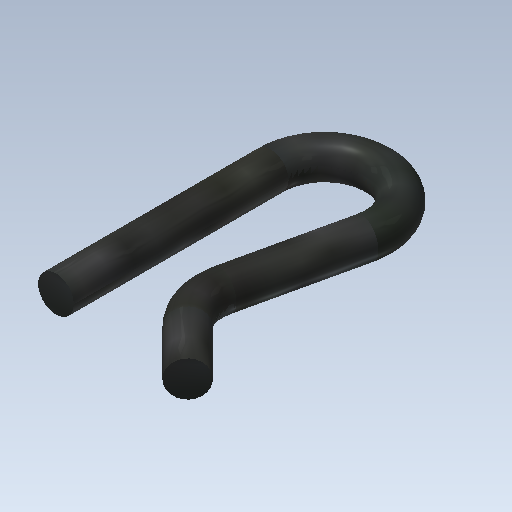
# Autodesk Inventor part: 500-177
Saved by Autodesk Inventor 2020 (Build 240168000, 168)
## iProperties
Created: 2015-04-18
Part Number: 500-177
Material: Steel
Document SubType Name: Modeling
Designer: Station9
Mass: 0.108858 g
Surface Area: 0.5704 cm^2
Volume: 0.0138673 cm^3
Density: 7.85 g/cm^3
Appearance: Plate
Author: Station9
Autodesk Inventor part; units mm, degrees
ref_plane "YZ Plane" through (0, 0, 0) normal (1, 0, 0) x (0, 1, 0)
ref_plane "XZ Plane" through (0, 0, 0) normal (0, 1, 0) x (-1, 0, 0)
ref_plane "XY Plane" through (0, 0, 0) normal (0, 0, 1) x (1, 0, 0)
sketch "Sketch1" plane through (0, 0, 0) normal (0, 1, 0) x (-1, 0, 0)
  line L0 (0, 0) -> (0, -6)
  arc A0 (-1.9758, -5.7812) -> (0, -6) centre (-1, -6) ccw
  line L1 (-1.9758, -5.7812) -> (-1.2485, -2.5376)
  line L2 (-1.7858, -0.6858) -> (-3.0444, 0.5729)
  arc A1 (-1.2485, -2.5376) -> (-1.7858, -0.6858) centre (-3.2, -2.1) ccw
  dimension "d0" = 2
  dimension "d1" = 1
  dimension "d2" = 6
  dimension "d3" = 1.78
  dimension "d4" = 3.9
  dimension "d5" = 2.2
  dimension "d6" = 45
  constraints: 6 end point, 4 point on circle, 4 tangent, 2 centre point, 1 vertical
  measures "d0" radius of A1
  measures "d1" radius of A0
  measures "d2" distance of L0.start L0.end
  measures "d3" distance of L2.start L2.end
  measures "d4" vertical distance of A0.centre A1.centre
  measures "d5" horizontal distance of A0.centre A1.centre
  measures "d6" angle of L0 L2
sketch "Sketch2" plane through (0, 0, 0) normal (0, 0, 1) x (1, 0, 0)
  circle A0 centre (-0.5, 0) radius 0.5
  point P0 (0, 0)
  point P1 (0, 0)
  dimension "d8" = 1
  dimension "d9" = 0.5
  constraints: 1 centre point
  measures "d8" diameter of A0
  measures "d9" distance of A0.centre point (0, 0)
sweep "Sweep1" add profiles "Sketch2" path "Sketch1"
body "Solid1"
